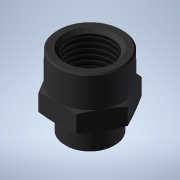
# Autodesk Inventor part: 8069220 NPFC-R-G14-G18-F
Saved by Autodesk Inventor 2021 (Build 250183000, 183)
## iProperties
Category: PARTsolutions
Company: FESTO
Created: 2026-09-15
Part Number: 8069220 NPFC-R-G14-G18-F
Material: Generic
Catalog Web Link: www.3dfindit.com
Description: NPFC-R-Threaded fittings
Vendor: FESTO
Document SubType Name: Modeling
Designer: psAdmin
Manufacturer: FESTO
Mass: 16 g
Surface Area: 18.8305 cm^2
Volume: 2.24605 cm^3
Density: 1 g/cm^3
Appearance: PSOLRGB-176-176-176
PSOL_IDENT_0: {$CADENAS_DATA/23d-libs/festo/parts/n/npfc/npfc_r.prj},190 {VTYP=3D},{NB=8069220 NPFC-R-G14-G18-F},{
PSOL_IDENT_1: LINA=8069220 NPFC-R-G14-G18-F},{NN=NPFC-R},{DATE=05.05.2026 12:08:01},{GEOMDATE=31.03.2025 12:44:06}
PSOL_IDENT_2: ,{VERSION=},{LINEID=1420},{WBVAR=},{WBNUMERIC=}  {NB=8069220 NPFC-R-G14-G18-F},{LINA=8069220 NPFC-R-
PSOL_IDENT_3: G14-G18-F},{KT=DUMMY},{TNR=8069220},{TYP=NPFC-R-G14-G18-F},{VERS=17},{D1=13.000},{D2=17.0},{T1=G1/8}
PSOL_IDENT_4: ,{T1C=9.728},{T2=G1/4},{T2C=13.157},{A=9.5},{A1=0.0},{A2=0.0},{B=19.00},{B1=6.00},{B2=8.00},{SW=17},
PSOL_IDENT_5: {CNSMASSEXACT=0.0160},{VERS2=3},{GTIN=4052568297589},{REACH=Ja},{REACHSVHC=Ja},{REACHHAZSUBS=7439-92
PSOL_IDENT_6: -1},{REACHSCIP=70f9d802-9488-43b2-bbff-53a39c1e9831,88e02f4a-9a81-4cf8-aaec-8b6ce5d79b8e},{REACHVALD
PSOL_IDENT_7: ATE=05.03.2025}
NB: 8069220 NPFC-R-G14-G18-F
NN: NPFC-R
NT: Threaded fittings
NBSYN: $TNR. $TYP.
LINA: 8069220 NPFC-R-G14-G18-F
CATALOG: Festo
TNR: 8069220
TYP: NPFC-R-G14-G18-F
D1: 13
D2: 17
T1: G1/8
T2: G1/4
A: 9.5
A1: 0
A2: 0
B: 19
B1: 6
B2: 8
SW: 17
CNSMASSEXACT: 0.016
GTIN: 4052568297589
REACH: Yes
REACHSVHC: Yes
REACHHAZSUBS: 7439-92-1
REACHSCIP: 70f9d802-9488-43b2-bbff-53a39c1e9831,88e02f4a-9a81-4cf8-aaec-8b6ce5d79b8e
REACHVALDATE: 05.03.2025
SUPPLIER: FESTO
ARTICLENO: 8069220 NPFC-R-G14-G18-F
BOMINFO: 8069220 NPFC-R-G14-G18-F
CREATOR: CADENAS GmbH
Title: 8069220 NPFC-R-G14-G18-F
Author: Cadenas PARTsolutions
Comments: Threaded fittings
Autodesk Inventor part; units mm, degrees
sketch "Sketch_12" plane through (0, 0, 0) normal (0, 0, 1) x (1, 0, 0)
  line L0 (0, 0) -> (0, 19)
  line L1 (0, 19) -> (8.1464, 19)
  line L2 (8.1464, 19) -> (8.5, 18.6464)
  line L3 (8.5, 18.6464) -> (8.5, 11)
  line L4 (8.5, 11) -> (10.2, 10.5445)
  line L5 (10.2, 10.5445) -> (10.2, 6.4555)
  line L6 (10.2, 6.4555) -> (8.5, 6)
  line L7 (8.5, 6) -> (6.5, 6)
  line L8 (6.5, 6) -> (6.5, 0.3536)
  line L9 (6.5, 0.3536) -> (6.1464, 0)
  line L10 (6.1464, 0) -> (0, 0)
  line L11 (0, 0) -> (0, 19)
  constraints: 24 end point
revolve "Revolution1" add sketch "Sketch_12" angle 360 about axis through (0, 0, 0) along (0, -1, 0)
sketch "Sketch_13" plane through (0, 0, 0) normal (0, 1, 0) x (-1, 0, 0)
  line L0 (17, 17) -> (-17, 17)
  line L1 (-17, 17) -> (-17, -17)
  line L2 (-17, -17) -> (17, -17)
  line L3 (17, -17) -> (17, 17)
  line L4 (9.815, 0) -> (4.9075, 8.5)
  line L5 (4.9075, 8.5) -> (-4.9075, 8.5)
  line L6 (-4.9075, 8.5) -> (-9.815, 0)
  line L7 (-9.815, 0) -> (-4.9075, -8.5)
  line L8 (-4.9075, -8.5) -> (4.9075, -8.5)
  line L9 (4.9075, -8.5) -> (9.815, 0)
  constraints: 20 end point
extrude "Extrusion1" cut sketch "Sketch_13" along normal blind 13.3
sketch "Sketch_14" plane through (0, 0, 0) normal (0, 0, 1) x (1, 0, 0)
  line L0 (0, 0) -> (0, 19)
  line L1 (0, 19) -> (6.5785, 19)
  line L2 (6.5785, 19) -> (5.7225, 18.144)
  line L3 (5.7225, 18.144) -> (5.7225, 8.55)
  line L4 (5.7225, 8.55) -> (4.283, 7.6)
  line L5 (4.283, 7.6) -> (4.283, 0.581)
  line L6 (4.283, 0.581) -> (4.864, 0)
  line L7 (4.864, 0) -> (0, 0)
  line L8 (0, 0) -> (0, 19)
  constraints: 18 end point
revolve "Revolution2" cut sketch "Sketch_14" angle 360 about axis through (0, 0, 0) along (0, -1, 0)
thread "Thread1" size "G13.157x1.337" designation "G 1/4" standard "ISO Pipe Threads" length 8.644
thread "Thread2" size "G9.728x0.907" designation "G 1/8" standard "ISO Pipe Threads" full length
ref_plane "ANBAU_XY" through (0, 7.5, 0) normal (0, 1, 0) x (1, 0, 0)
ref_plane "ANBAU_YZ" through (0, 7.5, 0) normal (1, 0, 0) x (0, 0, -1)
ref_plane "ANBAU_ZX" through (0, 7.5, 0) normal (0, 0, -1) x (0, 1, 0)
ref_plane "DICHTRING_XY" through (0, 9.5, 0) normal (0, 1, 0) x (1, 0, 0)
ref_plane "DICHTRING_YZ" through (0, 9.5, 0) normal (1, 0, 0) x (0, 0, -1)
ref_plane "DICHTRING_ZX" through (0, 9.5, 0) normal (0, 0, -1) x (0, 1, 0)
ref_plane "IP1_XY" through (0, 19, 0) normal (0, -1, 0) x (1, 0, 0)
ref_plane "IP1_YZ" through (0, 19, 0) normal (1, 0, 0) x (0, 0, 1)
ref_plane "IP1_ZX" through (0, 19, 0) normal (0, 0, 1) x (0, -1, 0)
ref_plane "IP2_XY" through (0, 9.5, 0) normal (0, 1, 0) x (1, 0, 0)
ref_plane "IP2_YZ" through (0, 9.5, 0) normal (1, 0, 0) x (0, 0, -1)
ref_plane "IP2_ZX" through (0, 9.5, 0) normal (0, 0, -1) x (0, 1, 0)
body "Solid1"
